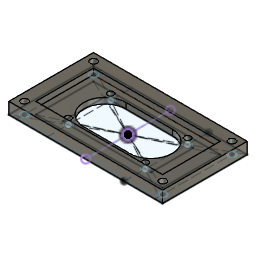
postolje v8 (Autodesk Fusion 360 design; units mm, degrees)
Autodesk Fusion 360 part; units mm, degrees
sketch "Sketch1" plane through (0, 0, 0) normal (0, 0, 1) x (1, 0, 0)
  line L0 (40, 22) -> (-40, 22)
  line L1 (-40, 22) -> (-40, -22)
  line L2 (-40, -22) -> (40, -22)
  line L3 (40, -22) -> (40, 22)
  line L4 (40, 22) -> (-40, -22) construction
  line L5 (-40, 22) -> (40, -22) construction
  line L6 (33, 15) -> (-33, 15)
  line L7 (-33, 15) -> (-33, -15)
  line L8 (-33, -15) -> (33, -15)
  line L9 (33, -15) -> (33, 15)
  line L10 (33, 15) -> (-33, -15) construction
  line L11 (-33, 15) -> (33, -15) construction
  line L12 (23, 11) -> (-23, 11)
  line L13 (-23, 11) -> (-23, -11)
  line L14 (-23, -11) -> (23, -11)
  line L15 (23, -11) -> (23, 11)
  line L16 (23, 11) -> (-23, -11) construction
  line L17 (-23, 11) -> (23, -11) construction
  line L18 (-40, 18.1224) -> (40, 18.1224) construction
  line L19 (-40, -17.8776) -> (40, -17.8776) construction
  line L20 (-36, 22) -> (-36, -22) construction
  line L21 (36, 22) -> (36, -22) construction
  circle A0 centre (-36, 18.1224) radius 1.8
  circle A1 centre (36, 18.1224) radius 1.8
  circle A2 centre (-36, -17.8776) radius 1.8
  circle A3 centre (36, -17.8776) radius 1.8
  line L22 (-20, 22) -> (-20, -22) construction
  line L23 (0, 22) -> (0, -22) construction
  line L24 (20, 22) -> (20, -22) construction
  dimension "d1" = 80
  dimension "d2" = 44
  dimension "d3" = 66
  dimension "d4" = 30
  dimension "d5" = 46
  dimension "d6" = 22
  dimension "d7" = 36
  dimension "d8" = 72
  dimension "d9" = 4
  dimension "d10" = 3.6
  dimension "d11" = 3.6
  dimension "d12" = 3.6
  dimension "d13" = 3.6
  dimension "d14" = 16
  constraint horizontal L0
  constraint perpendicular L0 L1
  constraint parallel L0 L2
  constraint parallel L1 L3
  constraint coincident L4 origin
  constraint coincident L5 origin
  constraint horizontal L6
  constraint perpendicular L6 L7
  constraint parallel L6 L8
  constraint parallel L7 L9
  constraint coincident L10 origin
  constraint coincident L11 origin
  constraint horizontal L12
  constraint perpendicular L12 L13
  constraint parallel L12 L14
  constraint parallel L13 L15
  constraint coincident L16 origin
  constraint coincident L17 origin
  constraint coincident L1 L18.start
  constraint coincident L3 L18.end
  constraint perpendicular L3 L18
  constraint coincident L1 L19.start
  constraint coincident L3 L19.end
  constraint perpendicular L3 L19
  constraint coincident L0 L20.start
  constraint coincident L2 L20.end
  constraint perpendicular L2 L20
  constraint coincident L0 L21.start
  constraint coincident L2 L21.end
  constraint perpendicular L2 L21
  constraint coincident L20 A0.centre
  constraint coincident L18 A0.centre
  constraint coincident L21 A1.centre
  constraint coincident L18 A1.centre
  constraint coincident L20 A2.centre
  constraint coincident L19 A2.centre
  constraint coincident L19 A3.centre
  constraint coincident L21 A3.centre
  constraint coincident L0 L22.start
  constraint coincident L2 L22.end
  constraint perpendicular L2 L22
  constraint midpoint L0 L23.start
  constraint midpoint L2 L23.end
  constraint symmetric L22.start L23 L24.start
  constraint symmetric L22.end L23 L24.end
  measures "d1" distance of L0.start L0.end
  measures "d2" distance of L0.start L2.end
  measures "d3" distance of L7.end L8.end
  measures "d4" distance of L6.end L7.end
  measures "d5" distance of L13.end L14.end
  measures "d6" distance of L12.end L13.end
  measures "d7" distance of L18 L19
  measures "d8" distance of L20 L21
  measures "d9" distance of L1 L20
  measures "d10" diameter of A0
  measures "d11" diameter of A1
  measures "d12" diameter of A2
  measures "d13" diameter of A3
  measures "d14" distance of L20 L22
sketch "Sketch2" plane through (0, 0, 0) normal (0, 0, 1) x (1, 0, 0)
extrude "Extrude1" add sketch "Sketch1" along normal blind 3 contours L6 L7 L8 L9
extrude "Extrude2" add sketch "Sketch1" along normal blind 6 contours L0 L1 L2 L3
fillet "Fillet1" radius 11 1 edges at (-23, 11, 1.5)
fillet "Fillet2" radius 11 1 edges at (23, 11, 1.5)
fillet "Fillet3" radius 11 1 edges at (23, -11, 1.5)
fillet "Fillet4" radius 11 1 edges at (-23, -11, 1.5)
sketch "Sketch3" plane through (0, 0, 0) normal (0, 0, 1) x (1, 0, 0)
  circle A0 centre (-20, 11) radius 1.6
  circle A1 centre (-20, -11) radius 1.6
  line L0 (0, 22) -> (0, -22)
  circle A2 centre (20, 11) radius 1.6
  circle A3 centre (20, -11) radius 1.6
  dimension "d29" = 3.2
  dimension "d30" = 3.2
  constraint symmetric A0 L0 A2
  constraint symmetric A1 L0 A3
  measures "d29" diameter of A0
  measures "d30" diameter of A1
extrude "Extrude3" cut sketch "Sketch3" along normal blind 12 contours A3
extrude "Extrude4" cut sketch "Sketch3" along normal blind 6 contours A2
extrude "Extrude5" cut sketch "Sketch3" along normal blind 8 contours A1
extrude "Extrude6" cut sketch "Sketch3" along normal blind 8 contours A0
